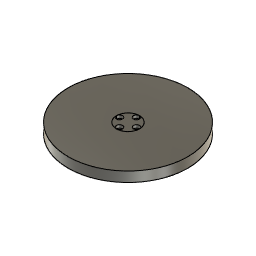
Baseplate_V1 (Autodesk Fusion 360 design; units mm, degrees)
Autodesk Fusion 360 part; units mm, degrees
sketch "Sketch1" plane through (0, 0, 0) normal (0, 0, 1) x (1, 0, 0) in component "Component"
  circle A0 centre (0, 0) radius 60
  circle A1 centre (0, 0) radius 11.5
  dimension "d1" = 120
  dimension "d2" = 23
  constraint coincident A0.centre A1.centre
  measures "d1" diameter of A0
  measures "d2" diameter of A1
extrude "Extrude1" add sketch "Sketch1" along normal blind 5 makes body 1 in component "Component"
sketch "Sketch1 (2)" plane through (0, 0, 5) normal (0, 0, 1) x (-1, 0, 0) in component "Component'"
  circle A0 centre (0, 0) radius 11.5
  circle A1 centre (0, 0) radius 60
  circle A2 centre (0, 0) radius 11.5
  constraint concentric A0 A2
extrude "Extrude1'" add sketch "Sketch1 (2)" along normal blind 2 separate body contours A0 A2 makes body 2 in component "Component'"
move_face "MoveFace1" to x (1, 0, 0) y (0, 1, 0) z (0, 0, 1) at (0, 0, -5) 1 faces at (-11.4857, 0.5732, 6.3333) on bodies 2 in component "Component'"
sketch "Sketch2" plane through (0, 0, 7) normal (0, 0, 1) x (-1, 0, 0) in component "Component'"
  circle A0 centre (0, 0) radius 11.5
sketch "Sketch1 (3)" plane through (0, 0, 7) normal (0, 0, 1) x (-1, 0, 0) in component "Component''"
  circle A0 centre (0, 0) radius 11.5
  circle A1 centre (8.5, 0) radius 1.5
  circle A2 centre (0, -8.5) radius 1.5
  circle A3 centre (-8.5, 0) radius 1.5
  circle A4 centre (0, 8.5) radius 1.5
  dimension "d7" = 23
  dimension "d8" = 3
  dimension "d9" = 3
  dimension "d10" = 3
  dimension "d11" = 3
  measures "d7" diameter of A0
  measures "d8" diameter of A1
  measures "d9" diameter of A2
  measures "d10" diameter of A3
  measures "d11" diameter of A4
extrude "Extrude2" cut sketch "Sketch1 (3)" against normal blind 4.5 contours A1 | A2 | A3 | A4 bodies 2 in component "Component'"
extrude "Extrude2'" add 1 faces at (43.5671, -3.5522, 5) along direction (0, 0, 1) blind 5 on bodies 1 bodies 1 in component "Component"
sketch "Sketch1 (4)" plane through (0, 0, 7) normal (0, 0, 1) x (-1, 0, 0) in component "Component'''"
  circle A0 centre (-8.5, 0) radius 2.5
  circle A1 centre (0, 8.5) radius 2.5
  circle A2 centre (8.5, 0) radius 2.5
  circle A3 centre (0, -8.5) radius 2.5
  dimension "d16" = 5
  dimension "d17" = 5
  dimension "d18" = 5
  dimension "d19" = 5
  measures "d16" diameter of A0
  measures "d17" diameter of A1
  measures "d18" diameter of A2
  measures "d19" diameter of A3
extrude "Extrude3" add sketch "Sketch2" along normal blind 3 bodies 2 in component "Component'"
extrude "Extrude4" cut sketch "Sketch1 (4)" along normal blind 7.5 bodies 2 in component "Component'"
hole "Hole1" at (-8.5, 0, 10) direction (0, 0, -1) diameter 6 depth 3 tip angle 180 bodies 2 in component "Component'"
hole "Hole2" at (0, -8.5, 10) direction (0, 0, -1) diameter 6 depth 3 tip angle 180 bodies 2 in component "Component'"
hole "Hole3" at (8.5, 0, 10) direction (0, 0, -1) diameter 6 depth 3 tip angle 180 bodies 2 in component "Component'"
hole "Hole4" at (0, 8.5, 10) direction (0, 0, -1) diameter 6 depth 3 tip angle 180 bodies 2 in component "Component'"
component "Component" placed x (1, 0, 0) y (0, 1, 0) z (0, 0, 1) at (0, 0, 0)
component "Component'" placed x (1, 0, 0) y (0, 1, 0) z (0, 0, 1) at (0, 0, 0)
component "Component''" placed x (1, 0, 0) y (0, 1, 0) z (0, 0, 1) at (0, 0, 0)
component "Component'''" placed x (1, 0, 0) y (0, 1, 0) z (0, 0, 1) at (0, 0, 0)
